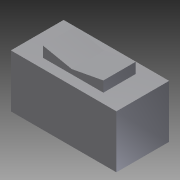
# Autodesk Inventor part: Switch
Saved by Autodesk Inventor 2012 (Build 160160000, 160)
## iProperties
Created: 2011-08-19
Part Number: Switch
Material: Default
Document SubType Name: Modeling
Designer: Minh Tran
Density: 1 g/cm^3
Author: Minh Tran
Autodesk Inventor part; units mm, degrees
ref_plane "YZ Plane" through (0, 0, 0) normal (1, 0, 0) x (0, 1, 0)
ref_plane "XZ Plane" through (0, 0, 0) normal (0, 1, 0) x (-1, 0, 0)
ref_plane "XY Plane" through (0, 0, 0) normal (0, 0, 1) x (1, 0, 0)
sketch "Sketch1" plane through (0, 0, 0) normal (0, 0, 1) x (1, 0, 0)
  line L0 (0, 0) -> (25.4, 0)
  line L1 (25.4, 0) -> (25.4, 12.7)
  line L2 (25.4, 12.7) -> (0, 12.7)
  line L3 (0, 12.7) -> (0, 0)
  dimension "d0" = 25.4
  dimension "d1" = 12.7
  constraints: 8 end point, 2 parallel, 1 horizontal, 1 perpendicular
  measures "d0" distance of L2.end L1.end
  measures "d1" distance of L1.end L0.end
extrude "Extrusion1" add sketch "Sketch1" along normal blind 12.7
sketch "Sketch2" plane through (0, 12.7, 0) normal (0, 1, 0) x (1, 0, 0)
  line L0 (5.398, -2.6368) -> (19.9399, -2.6368)
  line L1 (19.9399, -2.6368) -> (19.9399, -10.3739)
  line L2 (19.9399, -10.3739) -> (5.398, -10.3739)
  line L3 (5.398, -10.3739) -> (5.398, -2.6368)
  constraints: 8 end point, 2 parallel, 1 horizontal, 1 perpendicular
extrude "Extrusion2" add sketch "Sketch2" along normal blind 2.54
sketch "Sketch3" plane through (5.398, 12.7, 10.3739) normal (0, 0, 1) x (1, 0, 0)
  line L0 (14.5419, 2.54) -> (0, 2.54) projected
  line L1 (0, 2.54) -> (6.9268, 1.1079)
  line L2 (6.9268, 1.1079) -> (14.5419, 2.54)
  point P0 (-5.398, -12.7)
  constraints: 4 end point
extrude "Extrusion3" cut sketch "Sketch3" against normal blind 50.8
body "Solid1"
